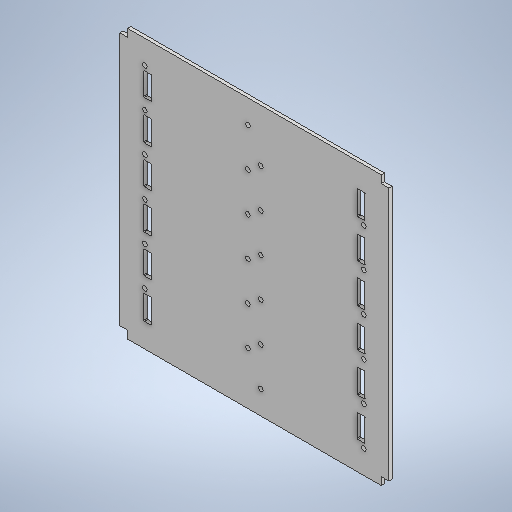
# Autodesk Inventor part: Baseplate_for_PCBs_v3_section
Saved by Autodesk Inventor 2025.1 (Build 291241000, 241)
## iProperties
Created: 2025-04-15
Part Number: Baseplate_for_PCBs_v3_section
Material: Generic
Document SubType Name: Modeling
Designer: edward.horrocks
Density: 1 g/cm^3
Appearance: Default
Author: edward.horrocks
Autodesk Inventor part; units mm, degrees
ref_plane "YZ Plane" through (0, 0, 0) normal (1, 0, 0) x (0, 1, 0)
ref_plane "XZ Plane" through (0, 0, 0) normal (0, 1, 0) x (-1, 0, 0)
ref_plane "XY Plane" through (0, 0, 0) normal (0, 0, 1) x (1, 0, 0)
sketch "Sketch2" plane through (0, 0, 0) normal (0, 0, 1) x (1, 0, 0)
  line L0 (-104.5, 104.5) -> (104.5, 104.5)
  line L1 (104.5, 104.5) -> (104.5, -104.5)
  line L2 (104.5, -104.5) -> (-104.5, -104.5)
  line L3 (-104.5, -104.5) -> (-104.5, 104.5)
  line L4 (-104.5, 104.5) -> (104.5, -104.5) construction
  line L5 (104.5, 104.5) -> (-104.5, -104.5) construction
  line L6 (-104.5, 104.5) -> (-98.5, 104.5)
  line L7 (-98.5, 104.5) -> (-98.5, 98.5)
  line L8 (-98.5, 98.5) -> (-104.5, 98.5)
  line L9 (-104.5, 98.5) -> (-104.5, 104.5)
  line L10 (104.5, 104.5) -> (98.5, 104.5)
  line L11 (98.5, 104.5) -> (98.5, 98.5)
  line L12 (98.5, 98.5) -> (104.5, 98.5)
  line L13 (104.5, 98.5) -> (104.5, 104.5)
  line L14 (104.5, -104.5) -> (98.5, -104.5)
  line L15 (98.5, -104.5) -> (98.5, -98.5)
  line L16 (98.5, -98.5) -> (104.5, -98.5)
  line L17 (104.5, -98.5) -> (104.5, -104.5)
  line L18 (-104.5, -104.5) -> (-98.5, -104.5)
  line L19 (-98.5, -104.5) -> (-98.5, -98.5)
  line L20 (-98.5, -98.5) -> (-104.5, -98.5)
  line L21 (-104.5, -98.5) -> (-104.5, -104.5)
  line L22 (-90, 90) -> (90, -90) construction
  line L23 (90, 90) -> (-90, -90) construction
  point P0 (0, 0)
  point P1 (-98.5, -104.5)
  point P2 (98.5, -104.5)
  point P3 (104.5, -98.5)
  point P4 (104.5, 98.5)
  point P5 (98.5, 104.5)
  point P6 (-98.5, 104.5)
  dimension "d0" = 209
  dimension "d1" = 209
  dimension "d2" = 6
  dimension "d3" = 6
  dimension "d4" = 6
  dimension "d5" = 6
  dimension "d6" = 6
  dimension "d7" = 6
  dimension "d8" = 6
  dimension "d9" = 6
  constraints: 48 end point, 10 parallel, 5 horizontal, 5 perpendicular, 4 midpoint
  measures "d0" distance of L1.end L2.end
  measures "d1" distance of L0.end L1.end
  measures "d2" distance of L7.end L8.end
  measures "d3" distance of L6.end L7.end
  measures "d4" distance of L12.end L11.end
  measures "d5" distance of L11.end L10.end
  measures "d6" distance of L15.end L16.end
  measures "d7" distance of L14.end L15.end
  measures "d8" distance of L20.end L19.end
  measures "d9" distance of L19.end L18.end
extrude "Extrusion1" add sketch "Sketch2" along normal blind 2.5 contours L0 L11 L12 L1 L16 L15 L2 L19 L20 L3 L8 L7
sketch "Sketch3" plane through (0, 0, 2.5) normal (0, 0, 1) x (1, 0, 0)
  circle A0 centre (-85, 86.25) radius 1.825
  point P0 (0, 0)
  dimension "d18" = 3.65
  constraints: 1 centre point
  measures "d18" diameter of A0
hole "Hole1" at (-85, 86.25, 2.5) direction (0, 0, -1) diameter 3.6 depth 10
pattern_linear "Rectangular Pattern1" count 2 spacing 80 along (1, 0, 0) count 6 spacing 30 along (0, -1, 0) of "Hole1"
sketch "Sketch4" plane through (0, 0, 2.5) normal (0, 0, 1) x (1, 0, 0)
  circle A0 centre (5, 63.75) radius 1.8
  line L0 (98.5, 104.5) -> (-98.5, 104.5) projected
  circle A1 centre (-5, 86.25) radius 1.8 projected
  point P0 (0, 0)
  dimension "d33" = 3.6
  dimension "d47" = 40.75
  dimension "d51" = 10
  constraints: 1 centre point
  measures "d33" diameter of A0
  measures "d47" distance from line of L0 A0.centre
  measures "d51" horizontal distance of A1.centre A0.centre
hole "Hole2" at (5, 63.75, 2.5) direction (0, 0, -1) diameter 3.6 depth 10
pattern_linear "Rectangular Pattern2" count 2 spacing 80 along (1, 0, 0) count 6 spacing 30 along (0, -1, 0) of "Hole2"
sketch "Sketch5" plane through (0, 0, 2.5) normal (0, 0, 1) x (1, 0, 0)
  line L0 (-85.348, 82.55) -> (-80.348, 82.55)
  line L1 (-79.848, 82.05) -> (-79.848, 65.05)
  line L2 (-80.348, 64.55) -> (-85.348, 64.55)
  line L3 (-85.848, 65.05) -> (-85.848, 82.05)
  circle A0 centre (-85, 86.25) radius 1.8 projected
  line L4 (-85.348, 52.79) -> (-80.348, 52.79)
  line L5 (-79.848, 52.29) -> (-79.848, 34.5)
  line L6 (-80.348, 34) -> (-85.348, 34)
  line L7 (-85.848, 34.5) -> (-85.848, 52.29)
  circle A1 centre (-85, 56.25) radius 1.8 projected
  arc A2 (-79.848, 82.05) -> (-80.348, 82.55) centre (-80.348, 82.05) ccw
  arc A3 (-85.348, 82.55) -> (-85.848, 82.05) centre (-85.348, 82.05) ccw
  arc A4 (-85.848, 65.05) -> (-85.348, 64.55) centre (-85.348, 65.05) ccw
  arc A5 (-80.348, 64.55) -> (-79.848, 65.05) centre (-80.348, 65.05) ccw
  arc A6 (-79.848, 52.29) -> (-80.348, 52.79) centre (-80.348, 52.29) ccw
  arc A7 (-80.348, 34) -> (-79.848, 34.5) centre (-80.348, 34.5) ccw
  arc A8 (-85.848, 34.5) -> (-85.348, 34) centre (-85.348, 34.5) ccw
  arc A9 (-85.348, 52.79) -> (-85.848, 52.29) centre (-85.348, 52.29) ccw
  point P0 (0, 0)
  point P1 (-85.848, 82.55)
  point P2 (-79.848, 64.55)
  point P3 (-79.848, 82.55)
  point P4 (-85.848, 64.55)
  point P5 (-85.848, 52.79)
  point P6 (-79.848, 34)
  point P7 (-79.848, 52.79)
  point P8 (-85.848, 34)
  dimension "d52" = 6
  dimension "d53" = 18
  dimension "d54" = 3.7
  dimension "d55" = 0.848
  dimension "d56" = 6
  dimension "d57" = 18.79
  dimension "d58" = 3.46
  dimension "d59" = 0.848
  dimension "d78" = 0.5
  constraints: 16 end point, 16 point on circle, 16 point on line, 16 tangent, 8 centre point, 7 equal radius, 4 parallel, 2 horizontal, 2 perpendicular
  measures "d52" distance of point (-79.848, 64.55) point (-85.848, 64.55)
  measures "d53" distance of point (-79.848, 82.55) point (-79.848, 64.55)
  measures "d54" distance from line of L0 A0.centre
  measures "d55" distance from line of A0.centre L3
  measures "d56" distance of point (-79.848, 34) point (-85.848, 34)
  measures "d57" distance of point (-79.848, 52.79) point (-79.848, 34)
  measures "d58" distance from line of L4 A1.centre
  measures "d59" distance from line of L7 A1.centre
  measures "d78" radius of A2
extrude "Extrusion2" cut sketch "Sketch5" against normal blind 10 contours L0 A2 L1 A5 L2 A4 L3 A3 | L4 A6 L5 A7 L6 A8 L7 A9
pattern_linear "Rectangular Pattern3" count 3 spacing 60 along (0, -1, 0) of "Extrusion2"
sketch "Sketch6" plane through (0, 0, 2.5) normal (0, 0, 1) x (1, 0, 0)
  line L0 (85.348, -82.55) -> (80.348, -82.55)
  line L1 (79.848, -82.05) -> (79.848, -65.05)
  line L2 (80.348, -64.55) -> (85.348, -64.55)
  line L3 (85.848, -65.05) -> (85.848, -82.05)
  circle A0 centre (85, -86.25) radius 1.8 projected
  line L4 (85.348, -52.79) -> (80.348, -52.79)
  line L5 (79.848, -52.29) -> (79.848, -34.5)
  line L6 (80.348, -34) -> (85.348, -34)
  line L7 (85.848, -34.5) -> (85.848, -52.29)
  circle A1 centre (85, -56.25) radius 1.8 projected
  arc A2 (85.348, -82.55) -> (85.848, -82.05) centre (85.348, -82.05) ccw
  arc A3 (85.848, -65.05) -> (85.348, -64.55) centre (85.348, -65.05) ccw
  arc A4 (80.348, -64.55) -> (79.848, -65.05) centre (80.348, -65.05) ccw
  arc A5 (79.848, -82.05) -> (80.348, -82.55) centre (80.348, -82.05) ccw
  arc A6 (85.348, -52.79) -> (85.848, -52.29) centre (85.348, -52.29) ccw
  arc A7 (85.848, -34.5) -> (85.348, -34) centre (85.348, -34.5) ccw
  arc A8 (80.348, -34) -> (79.848, -34.5) centre (80.348, -34.5) ccw
  arc A9 (79.848, -52.29) -> (80.348, -52.79) centre (80.348, -52.29) ccw
  point P0 (0, 0)
  point P1 (85.848, -82.55)
  point P2 (79.848, -64.55)
  point P3 (79.848, -82.55)
  point P4 (85.848, -64.55)
  point P5 (82.848, -82.55)
  point P6 (85.848, -52.79)
  point P7 (79.848, -34)
  point P8 (79.848, -52.79)
  point P9 (85.848, -34)
  dimension "d65" = 6
  dimension "d66" = 18
  dimension "d67" = 3.7
  dimension "d68" = 0.848
  dimension "d69" = 6
  dimension "d70" = 18.79
  dimension "d71" = 3.46
  dimension "d72" = 0.848
  dimension "d79" = 0.5
  constraints: 16 end point, 16 point on circle, 16 point on line, 16 tangent, 8 centre point, 7 equal radius, 4 parallel, 2 horizontal, 2 perpendicular, 1 midpoint
  measures "d65" distance of point (79.848, -64.55) point (85.848, -64.55)
  measures "d66" distance of point (79.848, -82.55) point (79.848, -64.55)
  measures "d67" vertical distance of point (82.848, -82.55) A0.centre
  measures "d68" distance from line of L3 A0.centre
  measures "d69" distance of point (79.848, -34) point (85.848, -34)
  measures "d70" distance of point (79.848, -52.79) point (79.848, -34)
  measures "d71" distance from line of L4 A1.centre
  measures "d72" distance from line of L7 A1.centre
  measures "d79" radius of A2
extrude "Extrusion3" cut sketch "Sketch6" against normal blind 10 contours L0 A5 L1 A4 L2 A3 L3 A2 | L4 A9 L5 A8 L6 A7 L7 A6
pattern_linear "Rectangular Pattern4" count 3 spacing 60 along (0, 1, 0) of "Extrusion3"
body "Solid1"
